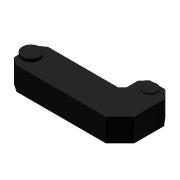
# Autodesk Inventor part: Bicep
Saved by Autodesk Inventor 2012 (Build 160160000, 160)
## iProperties
Created: 2013-02-21
Part Number: Bicep
Material: Default
Document SubType Name: Modeling
Designer: Andrew
Density: 1 g/cm^3
Author: Andrew
Autodesk Inventor part; units mm, degrees
ref_plane "YZ Plane" through (0, 0, 0) normal (1, 0, 0) x (0, 1, 0)
ref_plane "XZ Plane" through (0, 0, 0) normal (0, 1, 0) x (-1, 0, 0)
ref_plane "XY Plane" through (0, 0, 0) normal (0, 0, 1) x (1, 0, 0)
sketch "Sketch1" plane through (0, 0, 0) normal (0, 0, 1) x (1, 0, 0)
  arc A0 (2.8466, -52.6517) -> (4.2608, -52.0659) centre (2.8466, -50.6517) ccw
  line L0 (4.2608, -52.0659) -> (25.703, -30.6237)
  arc A1 (25.703, -30.6237) -> (26.2888, -29.2095) centre (24.2888, -29.2095) ccw
  line L1 (26.2888, -29.2095) -> (26.2888, 17.012)
  arc A2 (26.2888, 17.012) -> (25.8127, 18.3073) centre (24.2888, 17.012) ccw
  line L2 (25.8127, 18.3073) -> (13.9072, 32.3139)
  arc A3 (13.9072, 32.3139) -> (13.1317, 32.8733) centre (12.3833, 31.0186) ccw
  arc A4 (-11.6683, 32.8733) -> (-12.4438, 32.3139) centre (-10.9199, 31.0186) ccw
  line L3 (-12.4438, 32.3139) -> (-20.1922, 23.1981)
  arc A5 (-20.1922, 23.1981) -> (-20.6683, 21.9028) centre (-18.6683, 21.9028) ccw
  line L4 (-20.6683, 21.9028) -> (-20.6683, 4.4299)
  line L5 (-20.6683, 4.4299) -> (-27.2, -2.1017)
  arc A6 (-139.695, -52.3056) -> (-138.5704, -52.6517) centre (-138.5704, -50.6517) ccw
  arc A7 (-138.5704, -2.1017) -> (-139.695, -2.4479) centre (-138.5704, -4.1017) ccw
  line L6 (-139.695, -2.4479) -> (-143.4444, -4.9975)
  arc A8 (-143.4444, -4.9975) -> (-143.4828, -5.023) centre (-142.3581, -6.6767) ccw
  line L7 (-143.4828, -5.023) -> (-149.2963, -8.9767)
  line L8 (-149.2963, -8.9767) -> (-151.4209, -10.4215)
  arc A9 (-151.4209, -10.4215) -> (-152.2963, -12.0753) centre (-150.2963, -12.0753) ccw
  line L9 (-152.2963, -12.0753) -> (-152.2963, -12.6767)
  line L10 (-152.2963, -42.0767) -> (-152.2963, -42.6781)
  arc A10 (-152.2963, -42.6781) -> (-151.4209, -44.332) centre (-150.2963, -42.6781) ccw
  line L11 (-151.4209, -44.332) -> (-139.695, -52.3056)
  arc A11 (-5.1284, 30.1824) -> (-4.7861, 30.3893) centre (0.7317, 20.8733) ccw
  arc A12 (-148.0905, -39.6176) -> (-148.4375, -39.4185) centre (-141.2963, -27.3767) ccw
  line L12 (-11.6683, 32.8733) -> (13.1317, 32.8733)
  line L13 (-152.2963, -12.6767) -> (-152.2963, -18.7165)
  line L14 (-152.2963, -36.037) -> (-152.2963, -42.0767)
  line L15 (2.8466, -52.6517) -> (-138.5704, -52.6517)
  line L16 (-138.5704, -2.1017) -> (-27.2, -2.1017)
  circle A13 centre (0.7317, 20.8733) radius 11
  circle A14 centre (-141.2963, -27.3767) radius 14
  constraints: 10 end point, 3 tangent, 2 centre point, 2 concentric, 2 perpendicular, 2 point on circle, 1 coincident, 1 parallel
extrude "Extrusion1" add sketch "Sketch1" along normal mid plane 36.75 contours L15 A6 L11 A10 L10 L14 A12 A14 L13 L9 A9 L8 L7 A8 L6 A7 L16 L5 L4 A5 L3 A4 L12 A3 L2 A2 L1 A1 L0 A0
extrude "Extrusion2" add sketch "Sketch1" along normal mid plane 47 contours A12 A14
extrude "Extrusion3" add sketch "Sketch1" along normal mid plane 41 contours A13 A11
body "Solid1"
